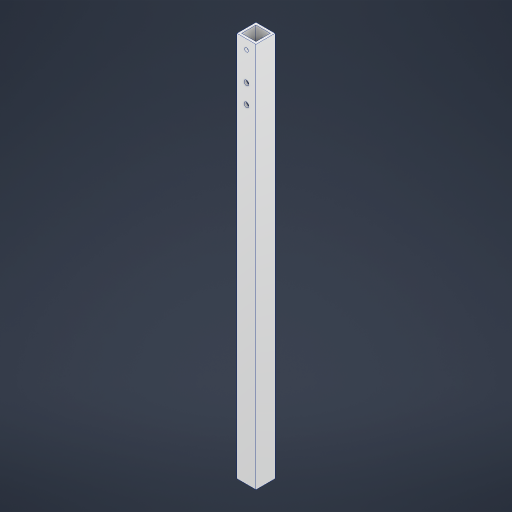
# Autodesk Inventor part: STRU_012_BilletPoleMiddle
Saved by Autodesk Inventor 2024.2 (Build 282272000, 272)
## iProperties
Created: 2024-07-25
Part Number: STRU_012_BilletPoleMiddle
Material: Aluminum 6061
Document SubType Name: Modeling
Designer: Bryan
Density: 2.7 g/cm^3
Appearance: Aluminum - Flat
Mass: 390.511 g
Surface Area: 920.312 cm^2
Volume: 144.634 cm^3
Author: Bryan
Autodesk Inventor part; units mm, degrees
ref_plane "YZ Plane" through (0, 0, 0) normal (1, 0, 0) x (0, 1, 0)
ref_plane "XZ Plane" through (0, 0, 0) normal (0, 1, 0) x (-1, 0, 0)
ref_plane "XY Plane" through (0, 0, 0) normal (0, 0, 1) x (1, 0, 0)
sketch "Sketch1" plane through (0, 0, 0) normal (0, 1, 0) x (-1, 0, 0)
  line L0 (-12.7, -12.7) -> (12.7, -12.7)
  line L1 (12.7, -12.7) -> (12.7, 12.7)
  line L2 (12.7, 12.7) -> (-12.7, 12.7)
  line L3 (-12.7, 12.7) -> (-12.7, -12.7)
  line L4 (-12.7, -12.7) -> (12.7, 12.7) construction
  line L5 (12.7, -12.7) -> (-12.7, 12.7) construction
  line L6 (9.525, 9.525) -> (9.525, -9.525)
  line L7 (9.525, -9.525) -> (-9.525, -9.525)
  line L8 (-9.525, -9.525) -> (-9.525, 9.525)
  line L9 (-9.525, 9.525) -> (9.525, 9.525)
  point P0 (0, 0)
  dimension "d0" = 25.4
  dimension "d1" = 25.4
  dimension "d2" = 3.175
  constraints: 20 end point, 4 parallel, 2 midpoint, 2 perpendicular, 1 horizontal, 3 other
  measures "d0" distance of L2.end L1.end
  measures "d1" distance of L1.end L0.end
  measures "d2" distance between parallel lines of L1 L6
extrude "Extrusion1" add sketch "Sketch1" along normal blind 514.35
sketch "Sketch4" plane through (-12.7, 0, 12.7) normal (0, 0, 1) x (1, 0, 0)
  line L0 (25.4, 488.95) -> (0, 488.95) construction
  line L1 (0, 488.95) -> (0, 514.35) construction
  line L2 (0, 514.35) -> (25.4, 514.35) construction
  line L3 (25.4, 514.35) -> (25.4, 488.95) construction
  line L4 (25.4, 488.95) -> (0, 514.35) construction
  line L5 (0, 488.95) -> (25.4, 514.35) construction
  circle A0 centre (12.7, 501.65) radius 2.4892
  circle A1 centre (12.7, 463.55) radius 3.2512
  circle A2 centre (12.7, 438.15) radius 3.2512
  point P0 (12.7, 0)
  dimension "d18" = 25.4
  dimension "d19" = 25.4
  dimension "d20" = 4.9784
  dimension "d21" = 6.5024
  dimension "d23" = 25.4
  dimension "d26" = 25.4
  constraints: 12 end point, 3 centre point, 2 coincident, 2 midpoint, 2 parallel, 2 vertical alignment, 1 equal radius, 1 horizontal, 1 perpendicular
  measures "d18" distance of L1.end L2.end
  measures "d19" distance of L0.end L1.end
  measures "d20" diameter of A0
  measures "d21" diameter of A1
  measures "d23" distance of A2.centre A1.centre
  measures "d26" distance from line of A1.centre L0
extrude "Extrusion4" cut sketch "Sketch4" against normal blind 25.4
body "Solid1"
